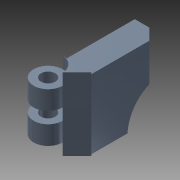
# Autodesk Inventor part: 夹具左
Saved by Autodesk Inventor 2015 (Build 190159000, 159)
## iProperties
Created: 2017-04-24
Part Number: 夹具左
Material: 常规
Document SubType Name: Modeling
Designer: Administrator
Density: 1 g/cm^3
Appearance: 钢蓝色
Author: Administrator
Autodesk Inventor part; units mm, degrees
ref_plane "YZ Plane" through (0, 0, 0) normal (1, 0, 0) x (0, 1, 0)
ref_plane "XZ Plane" through (0, 0, 0) normal (0, 1, 0) x (-1, 0, 0)
sketch "草图1" plane through (0, 0, 0) normal (0, 0, 1) x (1, 0, 0)
  arc A0 (0, 10) -> (10, 0) centre (0, 0) ccw
  circle A1 centre (0, 0) radius 5
  line L0 (0, 10) -> (20, 10)
  line L1 (20, 10) -> (20, 60)
  line L2 (20, 60) -> (0, 60)
  line L3 (0, 60) -> (0, 10)
  line L4 (10, 0) -> (20, 10)
  line L5 (10, 60) -> (20, 50)
  dimension "d0" = 20
  dimension "d1" = 10
  dimension "d2" = 20
  dimension "d3" = 50
  dimension "d4" = 135
  dimension "d5" = 10
  dimension "d6" = 45
  constraints: 12 end point, 2 centre point, 2 coincident, 2 parallel, 2 point on circle, 2 point on line, 1 horizontal, 1 midpoint, 1 perpendicular
  measures "d0" diameter of A0
  measures "d1" diameter of A1
  measures "d2" distance of L2.end L1.end
  measures "d3" distance of L0.end L1.end
  measures "d4" angle of L1 L4
  measures "d5" distance of L1.end L5.end
  measures "d6" angle of L1 L5
extrude "拉伸1" add sketch "草图1" along normal blind 50 contours L0 L4 A0 | L3 L2 L5 L1 L0
ref_plane "工作平面1" through (0, 0, 25) normal (0, 0, 1) x (1, 0, 0)
sketch "草图3" plane through (0, 0, 25) normal (0, 0, 1) x (1, 0, 0)
  arc A0 (0, 10) -> (14, 35) centre (-15.3214, 35) ccw
  line L0 (14, 35) -> (0, 35)
  line L1 (0, 60) -> (0, 10) projected
  line L2 (0, 35) -> (0, 10)
  line L3 (10, 60) -> (0, 60) projected
  line L4 (27.0643, 35) -> (-22.3857, 35) projected
  point P0 (0, 0)
  dimension "d13" = 14
  dimension "d14" = 25
  constraints: 4 end point, 2 point on circle, 1 centre point, 1 collinear, 1 midpoint, 1 parallel, 1 perpendicular, 1 point on line
  measures "d13" distance of L0.start L0.end
  measures "d14" distance of L0.end L1.end
revolve "旋转1" cut sketch "草图3" angle 360 about axis through (0, 35, 25) along (-1, 0, 0)
sketch "草图4" plane through (0, 0, 50) normal (0, 0, 1) x (1, 0, 0)
  line L0 (0, 60) -> (2, 60)
  line L1 (2, 60) -> (2, 10)
  line L2 (2, 10) -> (0, 10)
  line L3 (0, 10) -> (0, 60)
  arc A0 (0, 10) -> (10, 0) centre (0, 0) ccw projected
  line L4 (20, 50) -> (10, 60) projected
  line L5 (2, 60) -> (12, 60)
  line L6 (12, 60) -> (12, 58)
  line L7 (12, 58) -> (2, 58)
  line L8 (2, 58) -> (2, 60)
  dimension "d16" = 2
  dimension "d17" = 2
  constraints: 16 end point, 4 parallel, 2 horizontal, 2 perpendicular, 1 point on line, 1 tangent
  measures "d16" distance of L1.end L2.end
  measures "d17" distance of L5.end L6.end
extrude "拉伸2" cut sketch "草图4" against normal blind 50
sketch "草图5" plane through (2, 58, 50) normal (0, 1, 0) x (1, 0, 0)
  line L0 (0, 0) -> (0, 50) projected
  line L1 (18, 0) -> (0, 0)
  line L2 (0, 0) -> (0, 1)
  line L3 (0, 1) -> (18, 1)
  line L4 (18, 1) -> (18, 0)
  line L5 (18, 50) -> (0, 50)
  line L6 (0, 50) -> (0, 49)
  line L7 (0, 49) -> (18, 49)
  line L8 (18, 49) -> (18, 50)
  point P0 (-2, 50)
  dimension "d20" = 1
  dimension "d21" = 1
  constraints: 16 end point, 4 parallel, 2 horizontal, 2 perpendicular, 2 point on line
  measures "d20" distance between parallel lines of L1 L3
  measures "d21" distance between parallel lines of L5 L7
extrude "拉伸3" cut sketch "草图5" against normal blind 48
sketch "草图6" plane through (2, 35, 25) normal (-1, 0, 0) x (0, 0, 1)
  circle A0 centre (-25, 25) radius 25
  line L0 (-25, -45) -> (-25, -25) projected
  line L1 (-5.542, 23) -> (-24, 23) projected
  point P0 (-25, -35)
  dimension "d24" = 50
  dimension "d25" = 2
  constraints: 1 centre point, 1 point on line
  measures "d24" diameter of A0
  measures "d25" distance from line of L1 A0.centre
extrude "拉伸4" cut sketch "草图6" against normal blind 20
sketch "草图7" plane through (0, 0, 0) normal (0, 1, 0) x (-1, 0, 0)
  line L0 (0, 50) -> (10, 50)
  line L1 (10, 50) -> (10, 42)
  line L2 (10, 42) -> (0, 42)
  line L3 (0, 42) -> (0, 50)
  line L4 (0, 0) -> (10, 0)
  line L5 (10, 0) -> (10, 8)
  line L6 (10, 8) -> (0, 8)
  line L7 (0, 8) -> (0, 0)
  line L8 (0, 0) -> (0, 50) projected
  line L9 (0, 21) -> (10, 21)
  line L10 (10, 21) -> (10, 29)
  line L11 (10, 29) -> (0, 29)
  line L12 (0, 29) -> (0, 21)
  line L13 (0, -10) -> (0, 60) projected
  dimension "d28" = 8
  dimension "d29" = 13
  dimension "d30" = 21
  dimension "d31" = 13
  dimension "d32" = 8
  dimension "d33" = 10
  dimension "d34" = 10
  dimension "d35" = 10
  constraints: 24 end point, 6 parallel, 3 horizontal, 3 perpendicular, 3 point on line
  measures "d28" distance between parallel lines of L4 L6
  measures "d29" distance between parallel lines of L6 L9
  measures "d30" distance between parallel lines of L6 L11
  measures "d31" distance between parallel lines of L2 L11
  measures "d32" distance between parallel lines of L2 L0
  measures "d33" distance of L5.end L6.end
  measures "d34" distance of L10.end L11.end
  measures "d35" distance of L0.start L0.end
revolve "旋转2" cut sketch "草图7" angle 360 about axis through (0, 0, -10) along (0, 0, 1)
